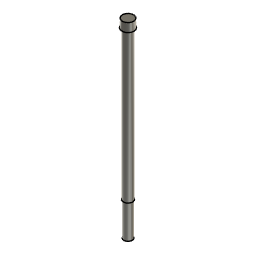
crystal_ball v29 (Autodesk Fusion 360 archive; units mm, degrees)
design "cane"
Autodesk Fusion 360 part; units mm, degrees
sketch "Sketch1" plane through (0, 0, 0) normal (0, 0, 1) x (1, 0, 0)
  circle A0 centre (0, 0) radius 6
  dimension "d1" = 12
  constraint coincident A0.centre origin
  measures "d1" diameter of A0
ref_plane "WorkPlane1" through (0, 0, -9) normal (0, 0, 1) x (1, 0, 0)
sketch "Sketch3" plane through (0, 0, -9) normal (0, 0, 1) x (1, 0, 0)
  circle A0 centre (0, 0) radius 6.5
  dimension "d8" = 13
  constraint coincident A0.centre origin
  measures "d8" diameter of A0
sketch "Sketch4" plane through (0, 0, -9) normal (0, 0, 1) x (1, 0, 0)
  circle A0 centre (0, 0) radius 5
  dimension "d9" = 10
  constraint coincident A0.centre origin
  measures "d9" diameter of A0
loft "Loft1" add profiles "Sketch3", "Sketch1" section 1 section 2
extrude "Extrude3" add sketch "Sketch4" against normal blind 160
sketch "Sketch5" plane through (0, 0, -169) normal (0, 0, -1) x (1, 0, 0)
  circle A0 centre (0, 0) radius 5
  circle A1 centre (0, 0) radius 4.5
  dimension "d12" = 9
  constraint concentric A0 A1
  measures "d12" diameter of A1
extrude "Extrude4" add sketch "Sketch5" along normal blind 36 contours A1
